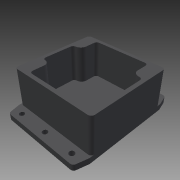
# Autodesk Inventor part: NEAMBox
Saved by Autodesk Inventor 2014 (Build 180170000, 170)
## iProperties
Created: 2015-04-18
Part Number: NEAMBox
Material: Generic
Document SubType Name: Modeling
Designer: Owner
Density: 1 g/cm^3
Appearance: Gray
Author: Owner
Autodesk Inventor part; units mm, degrees
ref_plane "YZ Plane" through (0, 0, 0) normal (1, 0, 0) x (0, 1, 0)
ref_plane "XZ Plane" through (0, 0, 0) normal (0, 1, 0) x (-1, 0, 0)
ref_plane "XY Plane" through (0, 0, 0) normal (0, 0, 1) x (1, 0, 0)
sketch "Sketch1" plane through (0, 0, 0) normal (0, 1, 0) x (-1, 0, 0)
  line L0 (-41.2899, 41.3823) -> (30.4199, 41.3823)
  line L1 (36.2591, 28.6823) -> (36.2591, -55.3155)
  line L2 (30.4199, -68.0155) -> (-41.2899, -68.0155)
  line L3 (-47.1291, -55.3155) -> (-47.1291, 28.6823)
  line L4 (-47.1291, 28.6823) -> (36.2591, 28.6823)
  line L5 (-47.1291, -55.3155) -> (36.2591, -55.3155)
  line L6 (36.2591, -55.3155) -> (33.4867, -65.6622)
  line L7 (-47.1291, -55.3155) -> (-44.3567, -65.6622)
  line L8 (-47.1291, 28.6823) -> (-44.3567, 39.0291)
  line L9 (36.2591, 28.6823) -> (33.4867, 39.0291)
  arc A0 (-44.3567, -65.6622) -> (-41.2899, -68.0155) centre (-41.2899, -64.8405) ccw
  arc A1 (30.4199, -68.0155) -> (33.4867, -65.6622) centre (30.4199, -64.8405) ccw
  arc A2 (33.4867, 39.0291) -> (30.4199, 41.3823) centre (30.4199, 38.2073) ccw
  arc A3 (-41.2899, 41.3823) -> (-44.3567, 39.0291) centre (-41.2899, 38.2073) ccw
  circle A4 centre (-35.4324, -61.0051) radius 2.5019
  circle A5 centre (24.5624, -61.0051) radius 2.5019
  circle A6 centre (-35.4324, 34.3719) radius 2.5019
  circle A7 centre (24.5624, 34.3719) radius 2.5019
  line L10 (-5.435, 41.3823) -> (-5.435, -68.0155) construction
  circle A8 centre (-5.435, 34.3719) radius 2.5019
  circle A9 centre (-5.435, -61.0051) radius 2.5019
  point P0 (0, 0)
  dimension "d2" = 12.7
  dimension "d3" = 12.7
  dimension "d4" = 15
  dimension "d5" = 15
  dimension "d6" = 15
  dimension "d7" = 83.3882
  dimension "d8" = 109.3978
  dimension "d9" = 3.175
  dimension "d10" = 7.0104
  dimension "d11" = 7.0104
  dimension "d12" = 7.0104
  dimension "d13" = 7.0104
  dimension "d14" = 59.9948
  dimension "d15" = 59.9948
  dimension "d16" = 5.0038
  dimension "d17" = 5.0038
  dimension "d18" = 5.0038
  dimension "d19" = 5.0038
  dimension "d20" = 29.9974
  dimension "d21" = 29.9974
  dimension "d42" = 5.0038
  dimension "d43" = 5.0038
  constraints: 22 end point, 10 centre point, 8 point on circle, 8 tangent, 3 equal radius, 3 parallel, 3 perpendicular, 2 midpoint, 2 point on line, 1 horizontal
  measures "d2" distance between parallel lines of L0 L4
  measures "d3" distance between parallel lines of L2 L5
  measures "d4" angle of L3 L8
  measures "d5" angle of L1 L9
  measures "d6" angle of L1 L6
  measures "d7" distance between parallel lines of L1 L3
  measures "d8" distance between parallel lines of L2 L0
  measures "d9" radius of A0
  measures "d10" distance from line of L0 A6.centre
  measures "d11" distance from line of L0 A7.centre
  measures "d12" distance from line of L2 A4.centre
  measures "d13" distance from line of L2 A5.centre
  measures "d14" distance of A5.centre A4.centre
  measures "d15" distance of A7.centre A6.centre
  measures "d16" diameter of A4
  measures "d17" diameter of A5
  measures "d18" diameter of A7
  measures "d19" diameter of A6
  measures "d20" distance from line of A7.centre L10
  measures "d21" distance from line of A5.centre L10
  measures "d42" diameter of A8
  measures "d43" diameter of A9
extrude "Extrusion1" add sketch "Sketch1" along normal blind 5.9944
sketch "Sketch2" plane through (0, 5.9944, 0) normal (0, 1, 0) x (1, 0, 0)
  line L0 (47.1291, -28.6823) -> (47.1291, 55.3155) projected
  line L1 (41.2899, 68.0155) -> (-30.4199, 68.0155) projected
  line L2 (-36.2591, 55.3155) -> (-36.2591, -28.6823) projected
  line L3 (-33.0841, 53.9185) -> (43.9541, 53.9185)
  line L4 (47.1291, 50.7435) -> (47.1291, -24.0849)
  line L5 (43.9541, -27.2599) -> (-33.0841, -27.2599)
  line L6 (-36.2591, -24.0849) -> (-36.2591, 50.7435)
  arc A0 (-36.2591, -24.0849) -> (-33.0841, -27.2599) centre (-33.0841, -24.0849) ccw
  arc A1 (43.9541, -27.2599) -> (47.1291, -24.0849) centre (43.9541, -24.0849) ccw
  arc A2 (47.1291, 50.7435) -> (43.9541, 53.9185) centre (43.9541, 50.7435) ccw
  arc A3 (-33.0841, 53.9185) -> (-36.2591, 50.7435) centre (-33.0841, 50.7435) ccw
  point P0 (0, 0)
  point P1 (-36.2591, 53.9185)
  point P2 (47.1291, -27.2599)
  dimension "d25" = 81.1784
  dimension "d26" = 14.097
  dimension "d27" = 3.175
  constraints: 8 end point, 8 point on circle, 8 tangent, 6 point on line, 4 centre point, 3 equal radius, 2 parallel, 1 horizontal, 1 perpendicular
  measures "d25" distance between parallel lines of L3 L5
  measures "d26" distance between parallel lines of L3 L1
  measures "d27" radius of A0
extrude "Extrusion2" add sketch "Sketch2" along normal blind 35.5092
sketch "Sketch3" plane through (0, 41.5036, 0) normal (0, 1, 0) x (1, 0, 0)
  line L0 (-36.2591, 50.7435) -> (-36.2591, -24.0849) projected
  line L1 (43.9541, 53.9185) -> (-33.0841, 53.9185) projected
  line L2 (43.1159, 26.9945) -> (43.1159, -0.3359)
  line L3 (-32.2459, -0.3359) -> (-32.2459, 26.9945)
  line L4 (-19.5713, 50.0069) -> (30.4413, 50.0069)
  line L5 (30.4413, -23.3483) -> (-19.5713, -23.3483)
  arc A0 (33.6163, 46.8319) -> (30.4413, 50.0069) centre (30.4413, 46.8319) ccw
  arc A1 (-19.5713, 50.0069) -> (-22.7463, 46.8319) centre (-19.5713, 46.8319) ccw
  arc A2 (-22.7463, -20.1733) -> (-19.5713, -23.3483) centre (-19.5713, -20.1733) ccw
  arc A3 (30.4413, -23.3483) -> (33.6163, -20.1733) centre (30.4413, -20.1733) ccw
  arc A4 (-32.2459, -0.3359) -> (-29.0709, -3.5109) centre (-29.0709, -0.3359) ccw
  arc A5 (-29.0709, 30.1695) -> (-32.2459, 26.9945) centre (-29.0709, 26.9945) ccw
  arc A6 (43.1159, 26.9945) -> (39.9409, 30.1695) centre (39.9409, 26.9945) ccw
  arc A7 (39.9409, -3.5109) -> (43.1159, -0.3359) centre (39.9409, -0.3359) ccw
  line L6 (33.6163, 46.8319) -> (33.6163, 36.5195)
  line L7 (33.6163, -9.8609) -> (33.6163, -20.1733)
  line L8 (-22.7463, -20.1733) -> (-22.7463, -9.8609)
  line L9 (-22.7463, 36.5195) -> (-22.7463, 46.8319)
  line L10 (39.9409, -3.5109) -> (39.9663, -3.5109)
  line L11 (-29.0963, -3.5109) -> (-29.0709, -3.5109)
  line L12 (-29.0709, 30.1695) -> (-29.0963, 30.1695)
  line L13 (39.9663, 30.1695) -> (39.9409, 30.1695)
  arc A8 (39.9663, -3.5109) -> (33.6163, -9.8609) centre (39.9663, -9.8609) ccw
  arc A9 (33.6163, 36.5195) -> (39.9663, 30.1695) centre (39.9663, 36.5195) ccw
  arc A10 (-29.0963, 30.1695) -> (-22.7463, 36.5195) centre (-29.0963, 36.5195) ccw
  arc A11 (-22.7463, -9.8609) -> (-29.0963, -3.5109) centre (-29.0963, -9.8609) ccw
  point P0 (0, 0)
  point P1 (43.1159, -3.5109)
  point P2 (43.1159, 30.1695)
  point P3 (-32.2459, -3.5109)
  point P4 (-22.7463, 50.0069)
  point P5 (33.6163, -23.3483)
  point P6 (33.6163, 50.0069)
  dimension "d30" = 56.3626
  dimension "d31" = 33.6804
  dimension "d32" = 73.3552
  dimension "d35" = 75.3618
  dimension "d36" = 4.0132
  dimension "d37" = 3.9116
  dimension "d38" = 3.175
  dimension "d39" = 6.35
  constraints: 32 tangent, 24 end point, 24 point on circle, 12 centre point, 10 equal radius, 10 parallel, 6 point on line, 4 perpendicular, 3 horizontal
  measures "d30" distance of point (-22.746, 50.007) point (33.616, 50.007)
  measures "d31" distance of point (43.116, 30.169) point (43.116, -3.511)
  measures "d32" distance of point (33.616, 50.007) point (33.616, -23.348)
  measures "d35" distance of point (43.116, -3.511) point (-32.246, -3.511)
  measures "d36" distance between parallel lines of L0 L3
  measures "d37" distance between parallel lines of L1 L4
  measures "d38" radius of A0
  measures "d39" radius of A8
extrude "Extrusion3" cut sketch "Sketch3" against normal blind 35.5092
body "Solid1"
